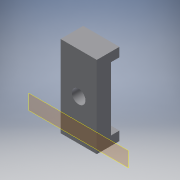
# Autodesk Inventor part: pulley_housing_top
Saved by Autodesk Inventor 2016 (Build 200138000, 138)
## iProperties
Created: 2016-05-29
Part Number: pulley_housing_top
Material: Generic
Document SubType Name: Modeling
Designer: ajar021
Density: 1 g/cm^3
Appearance: Default
Author: ajar021
Autodesk Inventor part; units mm, degrees
ref_plane "YZ Plane" through (0, 0, 0) normal (1, 0, 0) x (0, 1, 0)
ref_plane "XZ Plane" through (0, 0, 0) normal (0, 1, 0) x (-1, 0, 0)
ref_plane "XY Plane" through (0, 0, 0) normal (0, 0, 1) x (1, 0, 0)
ref_plane "Work Plane1" through (0, 69.5363, 0) normal (0, 0, 1) x (1, 0, 0)
sketch "Sketch1" plane through (0, 69.5363, 0) normal (0, 0, 1) x (1, 0, 0)
  line L0 (9.2773, 16.5681) -> (-0.7227, 16.5681) projected
  line L1 (0, -69.5363) -> (0, -2) projected
  line L2 (-20, 0) -> (-20, -2) projected
  line L3 (0, -2) -> (-20, -2)
  line L4 (-20, -2) -> (-20, 12)
  line L5 (-20, 12) -> (0, 12)
  line L6 (0, 12) -> (0, -2)
  dimension "d17" = 14
  dimension "d18" = 20
  constraints: 8 end point, 2 parallel, 1 horizontal, 1 perpendicular
  measures "d17" distance of L3.end L4.end
  measures "d18" distance of L1.end L3.end
extrude "Extrusion1" add sketch "Sketch1" along normal blind -3.1173
sketch "Sketch2" plane through (0, 69.5363, -3.1173) normal (0, 0, -1) x (1, 0, 0)
  line L0 (0, 2) -> (-20, -12)
  line L1 (-20, 2) -> (0, -12)
  circle A0 centre (-10, -5) radius 1.5
  point P0 (0, 69.5363)
  point P1 (-10, 4)
  dimension "d22" = 3
  constraints: 4 end point, 2 midpoint, 1 centre point
  measures "d22" diameter of A0
extrude "Extrusion2" cut sketch "Sketch2" against normal up to surface (3.1173 mm away)
sketch "Sketch3" plane through (0, 69.5363, -3.1173) normal (0, 0, -1) x (1, 0, 0)
  line L0 (0, -12) -> (0, 2) projected
  line L1 (-20, 2) -> (-20, -12) projected
  line L2 (-20, 2) -> (0, -12) construction
  line L3 (-20, -12) -> (0, 2) construction
  line L4 (-20, -12) -> (-20, -14.5)
  line L5 (-20, -14.5) -> (-17.5, -14.5)
  line L6 (0, 2) -> (0, 4.5)
  line L7 (0, 4.5) -> (-2.5, 4.5)
  line L8 (-20, -12) -> (0, -12) projected
  line L9 (-14, 22) -> (-6, 22)
  line L10 (-6, 22) -> (-6, -12)
  line L11 (-6, -12) -> (-14, -12)
  line L12 (-14, -12) -> (-14, 22)
  line L13 (-14, 22) -> (-6, -12) construction
  line L14 (-6, 22) -> (-14, -12) construction
  line L15 (-20, 2) -> (0, 2)
  line L16 (0, 2) -> (0, -12)
  line L17 (0, -12) -> (-20, -12)
  line L18 (-20, -12) -> (-20, 2)
  point P0 (0, 69.5363)
  point P1 (-10, 5)
  dimension "d7" = 2.5
  dimension "d8" = 2.5
  dimension "d9" = 2.5
  dimension "d10" = 2.5
  dimension "d28" = 8
  constraints: 32 end point, 4 parallel, 4 perpendicular, 4 point on line, 2 horizontal, 2 midpoint
  measures "d7" distance of L1.end L4.end
  measures "d8" distance of L4.end L5.end
  measures "d9" distance of L0.end L6.end
  measures "d10" distance of L6.end L7.end
  measures "d28" distance of L11.end L10.end
extrude "Extrusion4" cut sketch "Sketch3" against normal up to surface (3.1173 mm away) contours L8 L10 L15 L0 | L8 L1 L15 L12
sketch "Sketch4" plane through (-14, 67.5363, 0) normal (0, -1, 0) x (-1, 0, 0)
  line L0 (0, 0) -> (-8, 0)
  line L1 (-8, 0) -> (-8, 5)
  line L2 (-8, 5) -> (0, 5)
  line L3 (0, 5) -> (0, 0)
  point P0 (-14, 0)
  dimension "d34" = 5
  constraints: 8 end point, 2 parallel, 1 horizontal, 1 perpendicular
  measures "d34" distance of L0.end L1.end
extrude "Extrusion5" add sketch "Sketch4" along normal blind 2
sketch "Sketch5" plane through (-14, 81.5363, 0) normal (0, 1, 0) x (-1, 0, 0)
  line L0 (0, 0) -> (0, -5) projected
  line L1 (-8, 0) -> (0, 0)
  line L2 (0, 0) -> (0, -5)
  line L3 (0, -5) -> (-8, -5)
  line L4 (-8, -5) -> (-8, 0)
  dimension "d35" = 5
  constraints: 8 end point, 2 parallel, 1 horizontal, 1 perpendicular
  measures "d35" distance of L1.end L0.end
extrude "Extrusion6" add sketch "Sketch5" along normal blind 2
body "Solid1"
